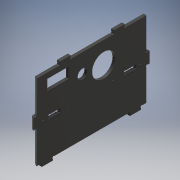
# Autodesk Inventor part: BA18
Saved by Autodesk Inventor 2017 (Build 210142000, 142)
## iProperties
Created: 2019-05-31
Part Number: BA18
Material: Polyethylene, High Density
Document SubType Name: Modeling
Designer: Dell
Density: 0.952 g/cm^3
Appearance: Smooth - Black
Mass: 274.487 g
Surface Area: 980.451 cm^2
Volume: 288.326 cm^3
Author: Dell
Autodesk Inventor part; units mm, degrees
ref_plane "YZ Plane" through (0, 0, 0) normal (1, 0, 0) x (0, 1, 0)
ref_plane "XZ Plane" through (0, 0, 0) normal (0, 1, 0) x (-1, 0, 0)
ref_plane "XY Plane" through (0, 0, 0) normal (0, 0, 1) x (1, 0, 0)
sketch "Sketch1" plane through (0, 0, 0) normal (0, 0, 1) x (1, 0, 0)
  line L0 (0, 0) -> (0, -195.6092) construction
  line L1 (0, -195.6092) -> (262.89, -347.3888) construction
  line L2 (262.89, -347.3888) -> (525.78, -195.6092) construction
  line L3 (525.78, -195.6092) -> (525.78, 0) construction
  line L4 (525.78, 0) -> (0, 0) construction
  line L5 (101.6, -254.268) -> (101.6, 0)
  line L6 (101.6, 0) -> (107.95, 0)
  line L7 (107.95, -257.9342) -> (101.6, -254.268)
  line L8 (107.95, 0) -> (107.95, -257.9342)
  point P0 (262.89, 0)
  dimension "d0" = 525.78
  dimension "d1" = 195.6092
  dimension "d2" = 120
  dimension "d3" = 6.35
  dimension "d4" = 101.6
  constraints: 18 end point, 4 point on line, 3 perpendicular, 1 collinear, 1 horizontal alignment, 1 midpoint, 1 parallel, 1 vertical, 1 vertical alignment
  measures "d0" distance of L3.end L0.start
  measures "d1" distance of L0.start L0.end
  measures "d2" angle of L2 L1
  measures "d3" distance between parallel lines of L5 L8
  measures "d4" distance between parallel lines of L0 L5
extrude "Extrusion1" add sketch "Sketch1" along normal blind 177.8
sketch "Sketch2" plane through (107.95, -257.9342, 0) normal (1, 0, 0) x (0, 0, -1)
  line L0 (0, 257.9342) -> (-177.8, 257.9342) projected
  line L1 (-101.6, 257.9342) -> (-76.2, 257.9342)
  line L2 (-76.2, 257.9342) -> (-76.2, 265.5542)
  line L3 (-76.2, 265.5542) -> (-101.6, 265.5542)
  line L4 (-101.6, 265.5542) -> (-101.6, 257.9342)
  line L5 (0, 3.6662) -> (-177.8, 3.6662) projected
  line L6 (-101.6, 3.6662) -> (-76.2, 3.6662)
  line L7 (-76.2, 3.6662) -> (-76.2, -7.62)
  line L8 (-76.2, -7.62) -> (-101.6, -7.62)
  line L9 (-101.6, -7.62) -> (-101.6, 3.6662)
  line L10 (0, 0) -> (-177.8, 0) projected
  point P0 (-88.9, 257.9342)
  point P1 (-88.9, 3.6662)
  dimension "d7" = 25.4
  dimension "d8" = 7.62
  dimension "d9" = 7.62
  constraints: 16 end point, 4 midpoint, 4 parallel, 2 horizontal, 2 perpendicular, 2 point on line, 1 vertical alignment
  measures "d7" distance of L3.end L2.end
  measures "d8" distance of L2.end L1.end
  measures "d9" distance between parallel lines of L8 L10
extrude "Extrusion2" add sketch "Sketch2" against normal blind 6.35
sketch "Sketch3" plane through (0, 0, 177.8) normal (0, 0, 1) x (1, 0, 0)
  line L0 (101.6, -254.268) -> (107.95, -257.9342) projected
  line L1 (107.95, -265.5542) -> (101.6, -265.5542) projected
  line L2 (107.95, -265.5542) -> (101.6, -261.888)
  line L3 (101.6, -265.5542) -> (101.6, -254.268) projected
  line L4 (101.6, -261.888) -> (101.6, -265.5542)
  point P0 (0, 0)
  constraints: 4 end point, 1 collinear, 1 parallel
extrude "Extrusion3" cut sketch "Sketch3" along normal through all both and the other way through all
sketch "Sketch4" plane through (101.6, -254.268, 0) normal (-1, 0, 0) x (0, 0, 1)
  line L0 (185.42, 203.468) -> (177.8, 203.468)
  line L1 (177.8, 203.468) -> (177.8, 178.068)
  line L2 (177.8, 178.068) -> (185.42, 178.068)
  line L3 (185.42, 178.068) -> (185.42, 203.468)
  line L4 (185.42, 76.468) -> (177.8, 76.468)
  line L5 (177.8, 76.468) -> (177.8, 51.068)
  line L6 (177.8, 51.068) -> (185.42, 51.068)
  line L7 (185.42, 51.068) -> (185.42, 76.468)
  line L8 (0, 254.268) -> (76.2, 254.268) projected
  line L9 (177.8, 254.268) -> (177.8, 0) projected
  dimension "d14" = 7.62
  dimension "d15" = 25.4
  dimension "d16" = 25.4
  dimension "d17" = 50.8
  dimension "d18" = 101.6
  constraints: 16 end point, 4 parallel, 2 horizontal, 2 perpendicular, 2 vertical alignment, 1 point on line
  measures "d14" distance of L0.start L0.end
  measures "d15" distance of L0.end L1.end
  measures "d16" distance of L4.end L5.end
  measures "d17" distance from line of L8 L0.end
  measures "d18" distance of L1.end L4.end
extrude "Extrusion4" add sketch "Sketch4" against normal blind 6.35
sketch "Sketch6" plane through (101.6, -254.268, 0) normal (-1, 0, 0) x (0, 0, 1)
  line L0 (165.1, 21.7338) -> (139.7, 21.7338)
  line L1 (139.7, 21.7338) -> (139.7, 72.5338)
  line L2 (139.7, 72.5338) -> (165.1, 72.5338)
  line L3 (165.1, 72.5338) -> (165.1, 21.7338)
  line L4 (101.6, -3.6662) -> (177.8, -3.6662) projected
  line L5 (177.8, 51.068) -> (177.8, 0) projected
  point P0 (0, 254.268)
  dimension "d21" = 25.4
  dimension "d22" = 50.8
  dimension "d23" = 25.4
  dimension "d24" = 12.7
  constraints: 8 end point, 2 parallel, 1 horizontal, 1 perpendicular
  measures "d21" distance of L1.end L2.end
  measures "d22" distance of L0.end L1.end
  measures "d23" distance between parallel lines of L4 L0
  measures "d24" distance between parallel lines of L5 L3
extrude "Extrusion5" cut sketch "Sketch6" against normal through all
sketch "Sketch7" plane through (101.6, -254.268, 0) normal (-1, 0, 0) x (0, 0, 1)
  line L0 (0, 0) -> (0, 254.268) projected
  line L1 (0, 216.168) -> (-7.62, 216.168)
  line L2 (-7.62, 216.168) -> (-7.62, 241.568)
  line L3 (-7.62, 241.568) -> (0, 241.568)
  line L4 (0, 241.568) -> (0, 216.168)
  line L5 (0, 9.0338) -> (-7.62, 9.0338)
  line L6 (-7.62, 9.0338) -> (-7.62, 34.4338)
  line L7 (-7.62, 34.4338) -> (0, 34.4338)
  line L8 (0, 34.4338) -> (0, 9.0338)
  line L9 (0, 254.268) -> (76.2, 254.268) projected
  line L10 (0, -3.6662) -> (76.2, -3.6662) projected
  dimension "d27" = 7.62
  dimension "d28" = 25.4
  dimension "d29" = 7.62
  dimension "d30" = 25.4
  dimension "d31" = 12.7
  dimension "d32" = 12.7
  constraints: 16 end point, 4 parallel, 2 horizontal, 2 perpendicular, 2 point on line
  measures "d27" distance of L2.end L3.end
  measures "d28" distance of L1.end L2.end
  measures "d29" distance of L6.end L7.end
  measures "d30" distance of L5.end L6.end
  measures "d31" distance between parallel lines of L9 L3
  measures "d32" distance between parallel lines of L5 L10
extrude "Extrusion6" add sketch "Sketch7" against normal blind 6.35
sketch "Sketch8" plane through (101.6, -254.268, 101.6) normal (-1, 0, 0) x (0, 0, 1)
  line L0 (-19.05, 203.468) -> (-12.7, 203.468)
  line L1 (-12.7, 203.468) -> (-12.7, 228.868)
  line L2 (-12.7, 228.868) -> (-19.05, 228.868)
  line L3 (-19.05, 228.868) -> (-19.05, 203.468)
  line L4 (-19.05, 25.668) -> (-12.7, 25.668)
  line L5 (-12.7, 25.668) -> (-12.7, 51.068)
  line L6 (-12.7, 51.068) -> (-19.05, 51.068)
  line L7 (-19.05, 51.068) -> (-19.05, 25.668)
  line L8 (-19.05, 38.368) -> (-19.05, 216.168) construction
  line L9 (0, 254.268) -> (76.2, 254.268) projected
  line L10 (76.2, 254.268) -> (76.2, 203.468) projected
  point P0 (-101.6, 254.268)
  dimension "d35" = 25.4
  dimension "d36" = 25.4
  dimension "d37" = 6.35
  dimension "d38" = 177.8
  dimension "d39" = 25.4
  dimension "d40" = 88.9
  constraints: 18 end point, 4 parallel, 2 horizontal, 2 midpoint, 2 perpendicular, 2 point on line
  measures "d35" distance of L6.end L4.start
  measures "d36" distance of L2.end L0.start
  measures "d37" distance of L4.start L4.end
  measures "d38" distance of L8.start L8.end
  measures "d39" distance from line of L9 L2.end
  measures "d40" distance between parallel lines of L1 L10
extrude "Extrusion7" cut sketch "Sketch8" against normal through all
sketch "Sketch9" plane through (101.6, -254.268, 101.6) normal (-1, 0, 0) x (0, 0, 1)
  line L0 (-19.05, 25.668) -> (-12.7, 25.668) projected
  line L1 (-15.875, 25.668) -> (-15.875, 0)
  line L2 (-19.05, 228.868) -> (-12.7, 228.868) projected
  line L3 (-15.875, 228.868) -> (-15.875, 254.268)
  line L4 (-15.875, 74.5009) -> (-15.875, 176.1009)
  line L5 (-12.7, 25.668) -> (-19.05, 25.668) projected
  circle A0 centre (-15.875, 12.834) radius 2.25
  circle A1 centre (-15.875, 74.5009) radius 2.25
  circle A2 centre (-15.875, 176.1009) radius 2.25
  circle A3 centre (-15.875, 241.568) radius 2.25
  line L6 (-101.6, 34.4338) -> (-101.6, 216.168) projected
  point P0 (-101.6, 254.268)
  point P1 (-25.4, 254.268)
  point P2 (-25.4, 0)
  point P3 (-101.6, 125.3009)
  point P4 (-15.875, 125.3009)
  dimension "d43" = 101.6
  dimension "d44" = 4.5
  dimension "d45" = 4.5
  dimension "d46" = 4.5
  dimension "d47" = 4.5
  constraints: 7 midpoint, 6 end point, 4 centre point, 3 horizontal alignment, 3 vertical, 2 coincident, 1 vertical alignment
  measures "d43" distance of L4.start L4.end
  measures "d44" diameter of A0
  measures "d45" diameter of A1
  measures "d46" diameter of A2
  measures "d47" diameter of A3
extrude "Extrusion8" cut sketch "Sketch9" against normal through all
sketch "Sketch10" plane through (101.6, -254.268, 101.6) normal (-1, 0, 0) x (0, 0, 1)
  circle A0 centre (31.75, 104.3058) radius 11.5
  line L0 (0, 254.268) -> (76.2, 254.268) projected
  line L1 (76.2, 178.068) -> (76.2, 76.468) projected
  point P0 (-101.6, 254.268)
  dimension "d50" = 23
  dimension "d51" = 149.9622
  dimension "d52" = 44.45
  constraints: 1 centre point
  measures "d50" diameter of A0
  measures "d51" distance from line of L0 A0.centre
  measures "d52" distance from line of L1 A0.centre
extrude "Extrusion9" cut sketch "Sketch10" against normal through all
sketch "Sketch11" plane through (107.95, 7.62, 101.6) normal (1, 0, 0) x (0, 0, -1)
  line L0 (11.43, -237.49) -> (20.32, -237.49)
  line L1 (20.32, -237.49) -> (20.32, -209.55)
  line L2 (20.32, -209.55) -> (11.43, -209.55)
  line L3 (11.43, -209.55) -> (11.43, -237.49)
  line L4 (11.43, -59.69) -> (20.32, -59.69)
  line L5 (20.32, -59.69) -> (20.32, -31.75)
  line L6 (20.32, -31.75) -> (11.43, -31.75)
  line L7 (11.43, -31.75) -> (11.43, -59.69)
  circle A0 centre (-31.75, -157.5822) radius 11.5 construction
  circle A1 centre (15.875, -85.7871) radius 2.25 construction
  circle A2 centre (15.875, -249.054) radius 2.25 construction
  circle A3 centre (15.875, -187.3871) radius 2.25 construction
  circle A4 centre (15.875, -20.32) radius 2.25 construction
  line L8 (12.7, -58.42) -> (12.7, -33.02) construction
  line L9 (12.7, -33.02) -> (19.05, -33.02) construction
  line L10 (19.05, -33.02) -> (19.05, -58.42) construction
  line L11 (19.05, -58.42) -> (12.7, -58.42) construction
  line L12 (12.7, -236.22) -> (12.7, -210.82) construction
  line L13 (12.7, -210.82) -> (19.05, -210.82) construction
  line L14 (19.05, -210.82) -> (19.05, -236.22) construction
  line L15 (19.05, -236.22) -> (12.7, -236.22) construction
  line L16 (-63.5, -240.1542) -> (-63.5, -189.3542) construction
  line L17 (-63.5, -189.3542) -> (-38.1, -189.3542) construction
  line L18 (-38.1, -189.3542) -> (-38.1, -240.1542) construction
  line L19 (-38.1, -240.1542) -> (-63.5, -240.1542) construction
  line L20 (101.6, -265.5542) -> (25.4, -265.5542) construction
  line L21 (101.6, -252.8542) -> (101.6, -265.5542) construction
  line L22 (101.6, -252.8542) -> (109.22, -252.8542) construction
  line L23 (109.22, -252.8542) -> (109.22, -227.4542) construction
  line L24 (109.22, -227.4542) -> (101.6, -227.4542) construction
  line L25 (101.6, -45.72) -> (101.6, -227.4542) construction
  line L26 (101.6, -45.72) -> (109.22, -45.72) construction
  line L27 (109.22, -45.72) -> (109.22, -20.32) construction
  line L28 (109.22, -20.32) -> (101.6, -20.32) construction
  line L29 (101.6, -7.62) -> (101.6, -20.32) construction
  line L30 (101.6, -7.62) -> (25.4, -7.62) construction
  line L31 (25.4, -7.62) -> (25.4, 0) construction
  line L32 (25.4, 0) -> (0, 0) construction
  line L33 (0, 0) -> (0, -7.62) construction
  line L34 (0, -7.62) -> (-76.2, -7.62) construction
  line L35 (-76.2, -58.42) -> (-76.2, -7.62) construction
  line L36 (-76.2, -58.42) -> (-83.82, -58.42) construction
  line L37 (-83.82, -58.42) -> (-83.82, -83.82) construction
  line L38 (-83.82, -83.82) -> (-76.2, -83.82) construction
  line L39 (-76.2, -185.42) -> (-76.2, -83.82) construction
  line L40 (-76.2, -185.42) -> (-83.82, -185.42) construction
  line L41 (-83.82, -185.42) -> (-83.82, -210.82) construction
  line L42 (-83.82, -210.82) -> (-76.2, -210.82) construction
  line L43 (-76.2, -265.5542) -> (-76.2, -210.82) construction
  line L44 (0, -265.5542) -> (-76.2, -265.5542) construction
  line L45 (0, -265.5542) -> (0, -273.1742) construction
  line L46 (0, -273.1742) -> (25.4, -273.1742) construction
  line L47 (25.4, -273.1742) -> (25.4, -265.5542) construction
  line L48 (13.6751, -235.2449) -> (18.0749, -235.2449)
  line L49 (18.0749, -235.2449) -> (18.0749, -211.7951)
  line L50 (18.0749, -211.7951) -> (13.6751, -211.7951)
  line L51 (13.6751, -211.7951) -> (13.6751, -235.2449)
  line L52 (13.6751, -57.4449) -> (18.0749, -57.4449)
  line L53 (18.0749, -57.4449) -> (18.0749, -33.9951)
  line L54 (18.0749, -33.9951) -> (13.6751, -33.9951)
  line L55 (13.6751, -33.9951) -> (13.6751, -57.4449)
  circle A5 centre (13.6751, -57.4449) radius 3.175
  circle A6 centre (13.6751, -33.9951) radius 3.175
  circle A7 centre (18.0749, -33.9951) radius 3.175
  circle A8 centre (18.0749, -57.4449) radius 3.175
  circle A9 centre (13.6751, -235.2449) radius 3.175
  circle A10 centre (13.6751, -211.7951) radius 3.175
  circle A11 centre (18.0749, -211.7951) radius 3.175
  circle A12 centre (18.0749, -235.2449) radius 3.175
  line L56 (-78.4451, -86.0651) -> (-86.0651, -86.0651) construction
  line L57 (-86.0651, -86.0651) -> (-86.0651, -56.1749) construction
  line L58 (-86.0651, -56.1749) -> (-78.4451, -56.1749) construction
  line L59 (-78.4451, -56.1749) -> (-78.4451, -5.3749) construction
  line L60 (-78.4451, -5.3749) -> (-2.2451, -5.3749) construction
  line L61 (-2.2451, -5.3749) -> (-2.2451, 2.2451) construction
  line L62 (-2.2451, 2.2451) -> (27.6451, 2.2451) construction
  line L63 (27.6451, 2.2451) -> (27.6451, -5.3749) construction
  line L64 (27.6451, -5.3749) -> (103.8451, -5.3749) construction
  line L65 (103.8451, -5.3749) -> (103.8451, -18.0749) construction
  line L66 (103.8451, -18.0749) -> (111.4651, -18.0749) construction
  line L67 (111.4651, -18.0749) -> (111.4651, -47.9651) construction
  line L68 (111.4651, -47.9651) -> (103.8451, -47.9651) construction
  line L69 (103.8451, -47.9651) -> (103.8451, -225.2091) construction
  line L70 (103.8451, -225.2091) -> (111.4651, -225.2091) construction
  line L71 (111.4651, -225.2091) -> (111.4651, -255.0993) construction
  line L72 (111.4651, -255.0993) -> (103.8451, -255.0993) construction
  line L73 (103.8451, -255.0993) -> (103.8451, -267.7993) construction
  line L74 (103.8451, -267.7993) -> (27.6451, -267.7993) construction
  line L75 (27.6451, -267.7993) -> (27.6451, -275.4193) construction
  line L76 (27.6451, -275.4193) -> (-2.2451, -275.4193) construction
  line L77 (-2.2451, -275.4193) -> (-2.2451, -267.7993) construction
  line L78 (-2.2451, -267.7993) -> (-78.4451, -267.7993) construction
  line L79 (-78.4451, -267.7993) -> (-78.4451, -213.0651) construction
  line L80 (-78.4451, -213.0651) -> (-86.0651, -213.0651) construction
  line L81 (-86.0651, -213.0651) -> (-86.0651, -183.1749) construction
  line L82 (-86.0651, -183.1749) -> (-78.4451, -183.1749) construction
  line L83 (-78.4451, -183.1749) -> (-78.4451, -86.0651) construction
  circle A13 centre (-78.4451, -213.0651) radius 3.175
  line L84 (-76.2, -185.42) -> (-83.82, -185.42) projected
  circle A14 centre (-78.4451, -183.1749) radius 3.175
  line L85 (-76.2, -185.42) -> (-76.2, -83.82) projected
  circle A15 centre (-78.4451, -86.0651) radius 3.175
  circle A16 centre (-78.4451, -56.1749) radius 3.175
  circle A17 centre (-2.2451, -5.3749) radius 3.175
  line L86 (101.6, -7.62) -> (25.4, -7.62) projected
  circle A18 centre (27.6451, -5.3749) radius 3.175
  circle A19 centre (103.8451, -18.0749) radius 3.175
  circle A20 centre (103.8451, -47.9651) radius 3.175
  circle A21 centre (103.8451, -225.2091) radius 3.175
  circle A22 centre (103.8451, -255.0993) radius 3.175
  circle A23 centre (27.6451, -267.7993) radius 3.175
  circle A24 centre (-2.2451, -267.7993) radius 3.175
  point P0 (12.7, -223.52)
  point P1 (11.43, -223.52)
  point P2 (12.7, -45.72)
  point P3 (11.43, -45.72)
  point P4 (15.875, -210.82)
  point P5 (15.875, -209.55)
  point P6 (15.875, -58.42)
  point P7 (15.875, -59.69)
  dimension "d58" = 6.35
  dimension "d59" = 6.35
  dimension "d60" = 6.35
  dimension "d55" = 1.27
  dimension "d56" = 1.27
  dimension "d57" = 1.27
  constraints: 88 end point, 20 coincident, 8 midpoint, 8 parallel, 4 perpendicular, 2 horizontal, 2 horizontal alignment, 2 vertical alignment, 1 point on line, 93 other
  measures "d55" distance between parallel lines of L3 L12
  measures "d56" distance between parallel lines of L2 L13
  measures "d57" distance between parallel lines of L11 L4
extrude "Extrusion10" cut sketch "Sketch11" against normal through all
sketch "Sketch12" plane through (101.6, -254.268, 101.6) normal (-1, 0, 0) x (0, 0, 1)
  circle A0 centre (24.75, 154.3058) radius 27.5
  circle A1 centre (31.75, 104.3058) radius 11.5 projected
  point P0 (-101.6, 254.268)
  dimension "d63" = 55
  dimension "d64" = 50
  dimension "d65" = 7
  constraints: 1 centre point
  measures "d63" diameter of A0
  measures "d64" vertical distance of A0.centre A1.centre
  measures "d65" horizontal distance of A0.centre A1.centre
extrude "Extrusion11" cut sketch "Sketch12" against normal through all contours A0
equation "\"d3\" = Panel_Thickness"
equation "\"d8\" = Panel_Thickness + Fit_Tolerance"
equation "\"d9\" = Panel_Thickness + Fit_Tolerance"
equation "\"d10\" = Panel_Thickness"
equation "\"d14\" = Panel_Thickness + Fit_Tolerance"
equation "\"d19\" = Panel_Thickness"
equation "\"d27\" = Panel_Thickness + Fit_Tolerance"
equation "\"d29\" = Panel_Thickness + Fit_Tolerance"
equation "\"d33\" = Panel_Thickness"
equation "\"d37\" = Panel_Thickness"
equation "\"d41\" = Panel_Thickness"
equation "\"d48\" = Panel_Thickness"
equation "\"d53\" = Panel_Thickness"
equation "\"d58\" = Tool_Dia"
equation "\"d59\" = Tool_Dia"
equation "\"d60\" = Tool_Dia"
equation "\"d55\" = Fit_Tolerance"
equation "\"d56\" = Fit_Tolerance"
equation "\"d57\" = Fit_Tolerance"
equation "\"d61\" = Panel_Thickness"
equation "\"Panel_Thickness\" = 6.35"
equation "\"Fit_Tolerance\" = 1.27"
equation "\"Tool_Dia\" = 6.35"
body "Solid1"
